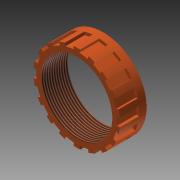
# Autodesk Inventor part: OBSN-30-B_ring
Saved by Autodesk Inventor 2013 (Build 170138000, 138)
## iProperties
Created: 2012-06-18
Part Number: OBSN-30-B_ring
Material: Nylon 6
Document SubType Name: Modeling
Designer: mstine
Density: 1 g/cm^3
Author: mstine
Autodesk Inventor part; units mm, degrees
ref_plane "YZ Plane" through (0, 0, 0) normal (1, 0, 0) x (0, 1, 0)
ref_plane "XZ Plane" through (0, 0, 0) normal (0, 1, 0) x (-1, 0, 0)
ref_plane "XY Plane" through (0, 0, 0) normal (0, 0, 1) x (1, 0, 0)
sketch "Sketch1" plane through (0, 0, 0) normal (0, 1, 0) x (-1, 0, 0)
  circle A0 centre (0, 0) radius 14.75
  circle A1 centre (0, 0) radius 18
  dimension "d0" = 29.5
  dimension "d1" = 36
  constraints: 2 centre point, 2 coincident
  measures "d0" diameter of A0
  measures "d1" diameter of A1
extrude "Extrusion1" add sketch "Sketch1" along normal blind 11
thread "Thread1" size "M30x1" class "6H" standard "ANSI Metric M Profile" full length
sketch "Sketch2" plane through (0, 0, 0) normal (0, -1, 0) x (1, 0, 0)
  circle A0 centre (0, 0) radius 14.75 projected
  line L0 (-18.761, 1.7111) -> (-16.7388, 1.7111)
  line L1 (-16.7388, 1.7111) -> (-16.7388, -1.7889)
  line L2 (-16.7388, -1.7889) -> (-18.761, -1.7889)
  line L3 (-18.761, -1.7889) -> (-18.761, 1.7111)
  line L4 (-18.2148, -4.8087) -> (-16.3145, -4.1171)
  line L5 (-16.3145, -4.1171) -> (-15.1175, -7.406)
  line L6 (-15.1175, -7.406) -> (-17.0177, -8.0976)
  line L7 (-17.0177, -8.0976) -> (-18.2148, -4.8087)
  line L8 (-15.4716, -10.7485) -> (-13.9225, -9.4487)
  line L9 (-13.9225, -9.4487) -> (-11.6728, -12.1298)
  line L10 (-11.6728, -12.1298) -> (-13.2219, -13.4297)
  line L11 (-13.2219, -13.4297) -> (-15.4716, -10.7485)
  line L12 (-10.8624, -15.3919) -> (-9.8512, -13.6406)
  line L13 (-9.8512, -13.6406) -> (-6.8202, -15.3906)
  line L14 (-6.8202, -15.3906) -> (-7.8313, -17.1419)
  line L15 (-7.8313, -17.1419) -> (-10.8624, -15.3919)
  line L16 (-4.9429, -18.1788) -> (-4.5918, -16.1873)
  line L17 (-4.5918, -16.1873) -> (-1.1449, -16.7951)
  line L18 (-1.1449, -16.7951) -> (-1.4961, -18.7866)
  line L19 (-1.4961, -18.7866) -> (-4.9429, -18.1788)
  line L20 (1.5727, -18.7731) -> (1.2215, -16.7816)
  line L21 (1.2215, -16.7816) -> (4.6684, -16.1738)
  line L22 (4.6684, -16.1738) -> (5.0195, -18.1653)
  line L23 (5.0195, -18.1653) -> (1.5727, -18.7731)
  line L24 (7.8986, -17.103) -> (6.8875, -15.3517)
  line L25 (6.8875, -15.3517) -> (9.9186, -13.6017)
  line L26 (9.9186, -13.6017) -> (10.9297, -15.353)
  line L27 (10.9297, -15.353) -> (7.8986, -17.103)
  line L28 (13.2719, -13.3701) -> (11.7228, -12.0703)
  line L29 (11.7228, -12.0703) -> (13.9725, -9.3891)
  line L30 (13.9725, -9.3891) -> (15.5216, -10.689)
  line L31 (15.5216, -10.689) -> (13.2719, -13.3701)
  line L32 (17.0443, -8.0246) -> (15.1441, -7.3329)
  line L33 (15.1441, -7.3329) -> (16.3411, -4.044)
  line L34 (16.3411, -4.044) -> (18.2414, -4.7356)
  line L35 (18.2414, -4.7356) -> (17.0443, -8.0246)
  line L36 (18.761, -1.7111) -> (16.7388, -1.7111)
  line L37 (16.7388, -1.7111) -> (16.7388, 1.7889)
  line L38 (16.7388, 1.7889) -> (18.761, 1.7889)
  line L39 (18.761, 1.7889) -> (18.761, -1.7111)
  line L40 (18.2148, 4.8087) -> (16.3145, 4.1171)
  line L41 (16.3145, 4.1171) -> (15.1175, 7.406)
  line L42 (15.1175, 7.406) -> (17.0177, 8.0976)
  line L43 (17.0177, 8.0976) -> (18.2148, 4.8087)
  line L44 (15.4716, 10.7485) -> (13.9225, 9.4487)
  line L45 (13.9225, 9.4487) -> (11.6728, 12.1298)
  line L46 (11.6728, 12.1298) -> (13.2219, 13.4297)
  line L47 (13.2219, 13.4297) -> (15.4716, 10.7485)
  line L48 (10.8624, 15.3919) -> (9.8512, 13.6406)
  line L49 (9.8512, 13.6406) -> (6.8202, 15.3906)
  line L50 (6.8202, 15.3906) -> (7.8313, 17.1419)
  line L51 (7.8313, 17.1419) -> (10.8624, 15.3919)
  line L52 (4.9429, 18.1788) -> (4.5918, 16.1873)
  line L53 (4.5918, 16.1873) -> (1.1449, 16.7951)
  line L54 (1.1449, 16.7951) -> (1.4961, 18.7866)
  line L55 (1.4961, 18.7866) -> (4.9429, 18.1788)
  line L56 (-1.5727, 18.7731) -> (-1.2215, 16.7816)
  line L57 (-1.2215, 16.7816) -> (-4.6684, 16.1738)
  line L58 (-4.6684, 16.1738) -> (-5.0195, 18.1653)
  line L59 (-5.0195, 18.1653) -> (-1.5727, 18.7731)
  line L60 (-7.8986, 17.103) -> (-6.8875, 15.3517)
  line L61 (-6.8875, 15.3517) -> (-9.9186, 13.6017)
  line L62 (-9.9186, 13.6017) -> (-10.9297, 15.353)
  line L63 (-10.9297, 15.353) -> (-7.8986, 17.103)
  line L64 (-13.2719, 13.3701) -> (-11.7228, 12.0703)
  line L65 (-11.7228, 12.0703) -> (-13.9725, 9.3891)
  line L66 (-13.9725, 9.3891) -> (-15.5216, 10.689)
  line L67 (-15.5216, 10.689) -> (-13.2719, 13.3701)
  line L68 (-17.0443, 8.0246) -> (-15.1441, 7.3329)
  line L69 (-15.1441, 7.3329) -> (-16.3411, 4.044)
  line L70 (-16.3411, 4.044) -> (-18.2414, 4.7356)
  line L71 (-18.2414, 4.7356) -> (-17.0443, 8.0246)
  dimension "d6" = 3.5
  dimension "d10" = 360
  constraints: 144 end point, 2 parallel, 1 horizontal, 1 perpendicular, 145 other
  measures "d6" distance of L2.end L0.start
extrude "Extrusion2" cut sketch "Sketch2" against normal blind 8 contours L0 L1 L2 L3 | L4 L5 L6 L7 | L8 L9 L10 L11 | L12 L13 L14 L15 | L16 L17 L18 L19 | L20 L21 L22 L23 | L24 L25 L26 L27 | L28 L29 L30 L31 | L32 L33 L34 L35 | L36 L37 L38 L39 | L40 L41 L42 L43 | L44 L45 L46 L47 | L48 L49 L50 L51 | L52 L53 L54 L55 | L56 L57 L58 L59 | L60 L61 L62 L63 | L64 L65 L66 L67 | L68 L69 L70 L71
body "Solid1"
